Autodesk Inventor part; units mm, degrees
(part 2 of 2)
  spline S316 degree 2 poles (54.544, 56.5341) (54.5622, 56.5549) (54.7827, 56.7857) knots 0 0 0 1 1 1
  spline S317 degree 2 poles (54.7827, 56.7857) (54.6633, 56.8583) (54.5622, 56.9751) (54.5622, 57.0477) knots 0 0 0 1 2 2 2
  spline S318 degree 2 poles (54.5622, 57.0477) (54.5622, 57.1281) (54.6945, 57.3486) (54.9357, 57.5509) knots 0 0 0 1 2 2 2
  spline S319 degree 2 poles (54.9124, 56.7676) (54.8008, 56.6482) (54.6893, 56.4433) (54.6893, 56.3577) knots 0 0 0 1 2 2 2
  spline S320 degree 2 poles (54.6893, 56.3577) (54.6893, 56.2462) (54.8242, 56.1632) knots 0 0 0 1 1 1
  spline S321 degree 2 poles (54.8242, 56.1632) (55.0602, 56.0179) (55.5038, 56.0179) knots 0 0 0 1 1 1
  spline S322 degree 2 poles (55.5038, 56.0179) (55.924, 56.0179) (56.3261, 56.3136) (56.3261, 56.4796) knots 0 0 0 1 2 2 2
  spline S323 degree 2 poles (56.3261, 56.4796) (56.3261, 56.6015) (56.2067, 56.6534) knots 0 0 0 1 1 1
  spline S324 degree 2 poles (56.2067, 56.6534) (56.0848, 56.7027) (55.7243, 56.7131) knots 0 0 0 1 1 1
  spline S325 degree 2 poles (55.7243, 56.7131) (55.1951, 56.7261) (54.9124, 56.7676) knots 0 0 0 1 1 1
  spline S326 degree 2 poles (55.343, 58.8635) (55.1692, 58.8635) (54.9357, 58.5885) (54.9357, 58.3032) knots 0 0 0 1 2 2 2
  spline S327 degree 2 poles (54.9357, 58.3032) (54.9357, 57.9322) (55.0939, 57.7299) knots 0 0 0 1 1 1
  spline S328 degree 2 poles (55.0939, 57.7299) (55.2159, 57.5743) (55.4052, 57.5743) knots 0 0 0 1 1 1
  spline S329 degree 2 poles (55.4052, 57.5743) (55.5816, 57.5743) (55.8125, 57.8415) (55.8125, 58.1268) knots 0 0 0 1 2 2 2
  spline S330 degree 2 poles (55.8125, 58.1268) (55.8125, 58.4977) (55.6516, 58.7078) knots 0 0 0 1 1 1
  spline S331 degree 2 poles (55.6516, 58.7078) (55.5323, 58.8635) (55.343, 58.8635) knots 0 0 0 1 1 1
  line L195 (60.0095, 57.3771) -> (59.7864, 56.7676)
  line L196 (59.7864, 56.7676) -> (57.9136, 56.7676)
  line L197 (57.9136, 56.7676) -> (57.9136, 56.8532)
  spline S332 degree 2 poles (57.9136, 56.8532) (58.741, 57.608) (59.4155, 58.5626) (59.4155, 58.9594) knots 0 0 0 1 2 2 2
  spline S333 degree 2 poles (59.4155, 58.9594) (59.4155, 59.2603) (59.0445, 59.6494) (58.7877, 59.6494) knots 0 0 0 1 2 2 2
  spline S334 degree 2 poles (58.7877, 59.6494) (58.5517, 59.6494) (58.1807, 59.3745) (58.09, 59.1099) knots 0 0 0 1 2 2 2
  line L198 (58.09, 59.1099) -> (58.0044, 59.1099)
  spline S335 degree 2 poles (58.0044, 59.1099) (58.064, 59.5431) (58.5465, 60.0074) (58.9096, 60.0074) knots 0 0 0 1 2 2 2
  spline S336 degree 2 poles (58.9096, 60.0074) (59.2961, 60.0074) (59.8149, 59.512) (59.8149, 59.1747) knots 0 0 0 1 2 2 2
  spline S337 degree 2 poles (59.8149, 59.1747) (59.8149, 58.9335) (59.7034, 58.6923) knots 0 0 0 1 1 1
  spline S338 degree 2 poles (59.7034, 58.6923) (59.5296, 58.3136) (59.1405, 57.8881) knots 0 0 0 1 1 1
  spline S339 degree 2 poles (59.1405, 57.8881) (58.5569, 57.2526) (58.4116, 57.1203) knots 0 0 0 1 1 1
  line L199 (58.4116, 57.1203) -> (59.2417, 57.1203)
  spline S340 degree 2 poles (59.2417, 57.1203) (59.4959, 57.1203) (59.6982, 57.1567) (59.8616, 57.2734) (59.9239, 57.3771) knots 0 0 0 1 2 3 3 3
  line L200 (59.9239, 57.3771) -> (60.0095, 57.3771)
  line L201 (62.3622, 60.0074) -> (62.3622, 59.9218)
  spline S341 degree 2 poles (62.3622, 59.9218) (62.0535, 59.8907) (61.6592, 59.7065) (61.2779, 59.3278) (61.0263, 58.8609) (60.9407, 58.5392) knots 0 0 0 1 2 3 4 4 4
  spline S342 degree 2 poles (60.9407, 58.5392) (61.2805, 58.7727) (61.6203, 58.7727) knots 0 0 0 1 1 1
  spline S343 degree 2 poles (61.6203, 58.7727) (61.9446, 58.7727) (62.4245, 58.2487) (62.4245, 57.8363) knots 0 0 0 1 2 2 2
  spline S344 degree 2 poles (62.4245, 57.8363) (62.4245, 57.4394) (62.1832, 57.11) knots 0 0 0 1 1 1
  spline S345 degree 2 poles (62.1832, 57.11) (61.8927, 56.7131) (61.4128, 56.7131) knots 0 0 0 1 1 1
  spline S346 degree 2 poles (61.4128, 56.7131) (61.0886, 56.7131) (60.8603, 56.9284) knots 0 0 0 1 1 1
  spline S347 degree 2 poles (60.8603, 56.9284) (60.4141, 57.346) (60.4141, 58.0152) knots 0 0 0 1 1 1
  spline S348 degree 2 poles (60.4141, 58.0152) (60.4141, 58.4407) (60.7565, 59.2085) (61.3921, 59.8025) (61.9757, 60.0074) (62.2273, 60.0074) knots 0 0 0 1 2 3 4 4 4
  line L202 (62.2273, 60.0074) -> (62.3622, 60.0074)
  spline S349 degree 2 poles (60.9018, 58.368) (60.8603, 58.0542) (60.8603, 57.8596) knots 0 0 0 1 1 1
  spline S350 degree 2 poles (60.8603, 57.8596) (60.8603, 57.6365) (61.0263, 57.11) (61.1897, 56.9543) knots 0 0 0 1 2 2 2
  spline S351 degree 2 poles (61.1897, 56.9543) (61.3116, 56.8454) (61.4829, 56.8454) knots 0 0 0 1 1 1
  spline S352 degree 2 poles (61.4829, 56.8454) (61.6852, 56.8454) (62.0068, 57.2293) (62.0068, 57.5847) knots 0 0 0 1 2 2 2
  spline S353 degree 2 poles (62.0068, 57.5847) (62.0068, 57.9841) (61.6878, 58.5678) (61.3947, 58.5678) knots 0 0 0 1 2 2 2
  spline S354 degree 2 poles (61.3947, 58.5678) (61.3065, 58.5678) (61.1015, 58.4925) (60.9018, 58.368) knots 0 0 0 1 2 2 2
  line L203 (63.3842, 59.6183) -> (63.3842, 58.9128)
  line L204 (63.3842, 58.9128) -> (63.8849, 58.9128)
  line L205 (63.8849, 58.9128) -> (63.8849, 58.7493)
  line L206 (63.8849, 58.7493) -> (63.3842, 58.7493)
  line L207 (63.3842, 58.7493) -> (63.3842, 57.3564)
  spline S355 degree 2 poles (63.3842, 57.3564) (63.3842, 57.1489) (63.5035, 57.0036) (63.5969, 57.0036) knots 0 0 0 1 2 2 2
  spline S356 degree 2 poles (63.5969, 57.0036) (63.6747, 57.0036) (63.8226, 57.0996) (63.8615, 57.193) knots 0 0 0 1 2 2 2
  line L208 (63.8615, 57.193) -> (63.9523, 57.193)
  spline S357 degree 2 poles (63.9523, 57.193) (63.8693, 56.9621) (63.5684, 56.7312) (63.4102, 56.7312) knots 0 0 0 1 2 2 2
  spline S358 degree 2 poles (63.4102, 56.7312) (63.3012, 56.7312) (63.0937, 56.8506) (62.9951, 57.0736) (62.9951, 57.3045) knots 0 0 0 1 2 3 3 3
  line L209 (62.9951, 57.3045) -> (62.9951, 58.7493)
  line L210 (62.9951, 58.7493) -> (62.6553, 58.7493)
  line L211 (62.6553, 58.7493) -> (62.6553, 58.8272)
  spline S359 degree 2 poles (62.6553, 58.8272) (62.785, 58.879) (63.0548, 59.1229) (63.1611, 59.2915) knots 0 0 0 1 2 2 2
  spline S360 degree 2 poles (63.1611, 59.2915) (63.2156, 59.3823) (63.3116, 59.6183) knots 0 0 0 1 1 1
  line L212 (63.3116, 59.6183) -> (63.3842, 59.6183)
  line L213 (64.7227, 60.0982) -> (64.7227, 58.5289)
  spline S361 degree 2 poles (64.7227, 58.5289) (64.9821, 58.8142) (65.2856, 58.975) (65.4386, 58.975) knots 0 0 0 1 2 2 2
  spline S362 degree 2 poles (65.4386, 58.975) (65.6202, 58.975) (65.8848, 58.7727) (65.947, 58.5574) knots 0 0 0 1 2 2 2
  spline S363 degree 2 poles (65.947, 58.5574) (65.9911, 58.4095) (65.9911, 58.0101) knots 0 0 0 1 1 1
  line L214 (65.9911, 58.0101) -> (65.9911, 57.2526)
  spline S364 degree 2 poles (65.9911, 57.2526) (65.9911, 57.0503) (66.0249, 56.9751) knots 0 0 0 1 1 1
  spline S365 degree 2 poles (66.0249, 56.9751) (66.0482, 56.918) (66.1598, 56.8532) (66.3102, 56.8532) knots 0 0 0 1 2 2 2
  line L215 (66.3102, 56.8532) -> (66.3102, 56.7676)
  line L216 (66.3102, 56.7676) -> (65.2545, 56.7676)
  line L217 (65.2545, 56.7676) -> (65.2545, 56.8532)
  line L218 (65.2545, 56.8532) -> (65.3037, 56.8532)
  spline S366 degree 2 poles (65.3037, 56.8532) (65.4542, 56.8532) (65.5709, 56.9439) (65.5943, 57.0321) knots 0 0 0 1 2 2 2
  spline S367 degree 2 poles (65.5943, 57.0321) (65.6021, 57.0711) (65.6021, 57.2526) knots 0 0 0 1 1 1
  line L219 (65.6021, 57.2526) -> (65.6021, 58.0101)
  spline S368 degree 2 poles (65.6021, 58.0101) (65.6021, 58.3628) (65.5294, 58.5833) (65.3712, 58.6923) (65.2571, 58.6923) knots 0 0 0 1 2 3 3 3
  spline S369 degree 2 poles (65.2571, 58.6923) (65.1429, 58.6923) (64.8965, 58.5704) (64.7227, 58.3862) knots 0 0 0 1 2 2 2
  line L220 (64.7227, 58.3862) -> (64.7227, 57.2526)
  spline S370 degree 2 poles (64.7227, 57.2526) (64.7227, 57.0321) (64.772, 56.9258) (64.9069, 56.8532) (65.0703, 56.8532) knots 0 0 0 1 2 3 3 3
  line L221 (65.0703, 56.8532) -> (65.0703, 56.7676)
  line L222 (65.0703, 56.7676) -> (64.0068, 56.7676)
  line L223 (64.0068, 56.7676) -> (64.0068, 56.8532)
  spline S371 degree 2 poles (64.0068, 56.8532) (64.1494, 56.8532) (64.2298, 56.8973) knots 0 0 0 1 1 1
  spline S372 degree 2 poles (64.2298, 56.8973) (64.2765, 56.9206) (64.3336, 57.0529) (64.3336, 57.2526) knots 0 0 0 1 2 2 2
  line L224 (64.3336, 57.2526) -> (64.3336, 59.1955)
  spline S373 degree 2 poles (64.3336, 59.1955) (64.3336, 59.5612) (64.2973, 59.7273) (64.2247, 59.7869) (64.165, 59.7869) knots 0 0 0 1 2 3 3 3
  spline S374 degree 2 poles (64.165, 59.7869) (64.1157, 59.7869) (64.0068, 59.7506) knots 0 0 0 1 1 1
  line L225 (64.0068, 59.7506) -> (63.973, 59.8362)
  line L226 (63.973, 59.8362) -> (64.6138, 60.0982)
  line L227 (64.6138, 60.0982) -> (64.7227, 60.0982)
  line L228 (69.7394, 57.3771) -> (69.5163, 56.7676)
  line L229 (69.5163, 56.7676) -> (67.6435, 56.7676)
  line L230 (67.6435, 56.7676) -> (67.6435, 56.8532)
  spline S375 degree 2 poles (67.6435, 56.8532) (68.471, 57.608) (69.1454, 58.5626) (69.1454, 58.9594) knots 0 0 0 1 2 2 2
  spline S376 degree 2 poles (69.1454, 58.9594) (69.1454, 59.2603) (68.7745, 59.6494) (68.5177, 59.6494) knots 0 0 0 1 2 2 2
  spline S377 degree 2 poles (68.5177, 59.6494) (68.2816, 59.6494) (67.9107, 59.3745) (67.8199, 59.1099) knots 0 0 0 1 2 2 2
  line L231 (67.8199, 59.1099) -> (67.7343, 59.1099)
  spline S378 degree 2 poles (67.7343, 59.1099) (67.7939, 59.5431) (68.2764, 60.0074) (68.6396, 60.0074) knots 0 0 0 1 2 2 2
  spline S379 degree 2 poles (68.6396, 60.0074) (69.0261, 60.0074) (69.5449, 59.512) (69.5449, 59.1747) knots 0 0 0 1 2 2 2
  spline S380 degree 2 poles (69.5449, 59.1747) (69.5449, 58.9335) (69.4333, 58.6923) knots 0 0 0 1 1 1
  spline S381 degree 2 poles (69.4333, 58.6923) (69.2595, 58.3136) (68.8704, 57.8881) knots 0 0 0 1 1 1
  spline S382 degree 2 poles (68.8704, 57.8881) (68.2868, 57.2526) (68.1415, 57.1203) knots 0 0 0 1 1 1
  line L232 (68.1415, 57.1203) -> (68.9716, 57.1203)
  spline S383 degree 2 poles (68.9716, 57.1203) (69.2258, 57.1203) (69.4281, 57.1567) (69.5916, 57.2734) (69.6538, 57.3771) knots 0 0 0 1 2 3 3 3
  line L233 (69.6538, 57.3771) -> (69.7394, 57.3771)
  spline S384 degree 2 poles (70.1129, 58.3369) (70.1129, 58.879) (70.4398, 59.6624) (70.7121, 59.8544) knots 0 0 0 1 2 2 2
  spline S385 degree 2 poles (70.7121, 59.8544) (70.9223, 60.0074) (71.1479, 60.0074) knots 0 0 0 1 1 1
  spline S386 degree 2 poles (71.1479, 60.0074) (71.5137, 60.0074) (71.8042, 59.6365) knots 0 0 0 1 1 1
  spline S387 degree 2 poles (71.8042, 59.6365) (72.1673, 59.1747) (72.1673, 58.3862) knots 0 0 0 1 1 1
  spline S388 degree 2 poles (72.1673, 58.3862) (72.1673, 57.8337) (71.8483, 57.0607) (71.3554, 56.7131) (71.1246, 56.7131) knots 0 0 0 1 2 3 3 3
  spline S389 degree 2 poles (71.1246, 56.7131) (70.6706, 56.7131) (70.3671, 57.25) knots 0 0 0 1 1 1
  spline S390 degree 2 poles (70.3671, 57.25) (70.1129, 57.7014) (70.1129, 58.3369) knots 0 0 0 1 1 1
  spline S391 degree 2 poles (70.5721, 58.2772) (70.5721, 57.6236) (70.7329, 57.2085) knots 0 0 0 1 1 1
  spline S392 degree 2 poles (70.7329, 57.2085) (70.8678, 56.8609) (71.1324, 56.8609) knots 0 0 0 1 1 1
  spline S393 degree 2 poles (71.1324, 56.8609) (71.2595, 56.8609) (71.5292, 57.0866) (71.5993, 57.3538) knots 0 0 0 1 2 2 2
  spline S394 degree 2 poles (71.5993, 57.3538) (71.7082, 57.7559) (71.7082, 58.4873) knots 0 0 0 1 1 1
  spline S395 degree 2 poles (71.7082, 58.4873) (71.7082, 59.0321) (71.5967, 59.3926) knots 0 0 0 1 1 1
  spline S396 degree 2 poles (71.5967, 59.3926) (71.5111, 59.6624) (71.3788, 59.774) knots 0 0 0 1 1 1
  spline S397 degree 2 poles (71.3788, 59.774) (71.2828, 59.8518) (71.1453, 59.8518) knots 0 0 0 1 1 1
  spline S398 degree 2 poles (71.1453, 59.8518) (70.9871, 59.8518) (70.8626, 59.7091) knots 0 0 0 1 1 1
  spline S399 degree 2 poles (70.8626, 59.7091) (70.694, 59.5146) (70.5721, 58.6819) (70.5721, 58.2772) knots 0 0 0 1 2 2 2
  line L234 (74.5382, 57.3771) -> (74.3151, 56.7676)
  line L235 (74.3151, 56.7676) -> (72.4423, 56.7676)
  line L236 (72.4423, 56.7676) -> (72.4423, 56.8532)
  spline S400 degree 2 poles (72.4423, 56.8532) (73.2698, 57.608) (73.9442, 58.5626) (73.9442, 58.9594) knots 0 0 0 1 2 2 2
  spline S401 degree 2 poles (73.9442, 58.9594) (73.9442, 59.2603) (73.5733, 59.6494) (73.3165, 59.6494) knots 0 0 0 1 2 2 2
  spline S402 degree 2 poles (73.3165, 59.6494) (73.0804, 59.6494) (72.7095, 59.3745) (72.6187, 59.1099) knots 0 0 0 1 2 2 2
  line L237 (72.6187, 59.1099) -> (72.5331, 59.1099)
  spline S403 degree 2 poles (72.5331, 59.1099) (72.5928, 59.5431) (73.0752, 60.0074) (73.4384, 60.0074) knots 0 0 0 1 2 2 2
  spline S404 degree 2 poles (73.4384, 60.0074) (73.8249, 60.0074) (74.3437, 59.512) (74.3437, 59.1747) knots 0 0 0 1 2 2 2
  spline S405 degree 2 poles (74.3437, 59.1747) (74.3437, 58.9335) (74.2321, 58.6923) knots 0 0 0 1 1 1
  spline S406 degree 2 poles (74.2321, 58.6923) (74.0583, 58.3136) (73.6692, 57.8881) knots 0 0 0 1 1 1
  spline S407 degree 2 poles (73.6692, 57.8881) (73.0856, 57.2526) (72.9403, 57.1203) knots 0 0 0 1 1 1
  line L238 (72.9403, 57.1203) -> (73.7704, 57.1203)
  spline S408 degree 2 poles (73.7704, 57.1203) (74.0246, 57.1203) (74.2269, 57.1567) (74.3904, 57.2734) (74.4526, 57.3771) knots 0 0 0 1 2 3 3 3
  line L239 (74.4526, 57.3771) -> (74.5382, 57.3771)
  line L240 (76.8209, 59.9426) -> (76.6393, 59.5457)
  line L241 (76.6393, 59.5457) -> (75.6848, 59.5457)
  line L242 (75.6848, 59.5457) -> (75.4746, 59.1203)
  spline S409 degree 2 poles (75.4746, 59.1203) (76.0946, 59.0295) (76.4577, 58.6586) knots 0 0 0 1 1 1
  spline S410 degree 2 poles (76.4577, 58.6586) (76.769, 58.3395) (76.769, 57.9089) knots 0 0 0 1 1 1
  spline S411 degree 2 poles (76.769, 57.9089) (76.769, 57.6599) (76.5641, 57.2319) (76.2554, 56.9336) (76.0661, 56.8428) knots 0 0 0 1 2 3 3 3
  spline S412 degree 2 poles (76.0661, 56.8428) (75.7963, 56.7131) (75.5135, 56.7131) knots 0 0 0 1 1 1
  spline S413 degree 2 poles (75.5135, 56.7131) (75.2256, 56.7131) (74.9662, 56.9076) (74.9662, 57.0244) knots 0 0 0 1 2 2 2
  spline S414 degree 2 poles (74.9662, 57.0244) (74.9662, 57.0892) (75.0726, 57.1904) (75.1556, 57.1904) knots 0 0 0 1 2 2 2
  spline S415 degree 2 poles (75.1556, 57.1904) (75.2152, 57.1904) (75.3086, 57.1515) (75.4176, 57.0736) knots 0 0 0 1 2 2 2
  spline S416 degree 2 poles (75.4176, 57.0736) (75.594, 56.9543) (75.7755, 56.9517) knots 0 0 0 1 1 1
  spline S417 degree 2 poles (75.7755, 56.9517) (76.0479, 56.9517) (76.4655, 57.3668) (76.4655, 57.6651) knots 0 0 0 1 2 2 2
  spline S418 degree 2 poles (76.4655, 57.6651) (76.4655, 57.953) (76.0946, 58.4536) (75.7678, 58.5885) knots 0 0 0 1 2 2 2
  spline S419 degree 2 poles (75.7678, 58.5885) (75.5135, 58.6949) (75.0726, 58.7104) knots 0 0 0 1 1 1
  line L243 (75.0726, 58.7104) -> (75.6822, 59.9426)
  line L244 (75.6822, 59.9426) -> (76.8209, 59.9426)
  point P0 (0, 120.8)
  dimension "d0" = 191.4
  dimension "d1" = 121.8
  constraints: 2 other
emboss "Emboss2" sketch "Sketch9" operation cut depth 1 direction (0, 1, 0)
sketch "Sketch10" plane through (0, 0, -120.8) normal (0, -1, 0) x (1, 0, 0)
  point P0 (0, 120.8)
sketch "Sketch11" plane through (0, 0, -120.8) normal (0, -1, 0) x (1, 0, 0)
  point P0 (0, 120.8)
sketch "Sketch13" plane through (110, 12.5, -116.4021) normal (1, 0, 0) x (0, 0, -1)
  point P0 (-116.4021, -12.5)
sketch "Sketch14" plane through (110, 12.5, -116.4021) normal (1, 0, 0) x (0, 0, -1)
  point P0 (-116.4021, -12.5)
ref_plane "Work Plane1" through (111, 12.5, -116.4021) normal (1, 0, 0) x (0, 0, -1)
sketch "Sketch16" plane through (111, 12.5, -116.4021) normal (1, 0, 0) x (0, 0, -1)
  arc A0 (-4, 14.7262) -> (-4, 9.7262) centre (-4, 12.2262) ccw
  line L0 (0, 178.9) -> (0, 0) projected
  line L1 (-4, 14.7262) -> (-4, 9.7262)
  point P0 (-116.4021, -12.5)
  dimension "d27" = 5
  dimension "d28" = 4
  constraints: 2 end point, 2 point on circle, 1 centre point, 1 vertical
  measures "d27" diameter of A0
  measures "d28" distance from line of A0.centre L0
revolve "Revolution2" cut sketch "Sketch16" angle 360 about axis through (111, 27.2262, -112.4021) along (0, -1, 0)
sketch "Sketch17" plane through (111, 12.5, -116.4021) normal (1, 0, 0) x (0, 0, -1)
  point P0 (-116.4021, -12.5)
sketch "Sketch18" plane through (111, 12.5, -116.4021) normal (1, 0, 0) x (0, 0, -1)
  arc A0 (-107.0042, 14.736) -> (-107.0042, 9.736) centre (-107.0042, 12.236) ccw
  line L0 (-111.0042, 178.9) -> (-111.0042, 0) projected
  line L1 (-111.0042, 0) -> (-104.0021, 0) projected
  line L2 (-107.0042, 14.736) -> (-107.0042, 9.736)
  point P0 (-116.4021, -12.5)
  dimension "d30" = 5
  dimension "d31" = 4
  dimension "d32" = 12.236
  constraints: 2 end point, 2 point on circle, 1 centre point, 1 parallel
  measures "d30" diameter of A0
  measures "d31" distance from line of A0.centre L0
  measures "d32" distance from line of A0.centre L1
revolve "Revolution3" cut sketch "Sketch18" angle 360 about axis through (111, 27.236, -9.3979) along (0, -1, 0)
sketch "Sketch19" plane through (110, 12.5, -116.4021) normal (1, 0, 0) x (0, 0, -1)
  point P0 (-116.4021, -12.5)
sketch "Sketch20" plane through (110, 12.5, -116.4021) normal (1, 0, 0) x (0, 0, -1)
  line L0 (-104.0021, 166.4) -> (-7.0021, 166.4) projected
  line L1 (-104.0021, 0) -> (-104.0021, 178.9) projected
  line L2 (-7.0021, 166.4) -> (-104.0021, 166.4)
  line L3 (-104.0021, 166.4) -> (-104.0021, 168.4)
  line L4 (-104.0021, 168.4) -> (-7.0021, 168.4)
  line L5 (-7.0021, 168.4) -> (-7.0021, 166.4)
  point P0 (-116.4021, -12.5)
  dimension "d34" = 2
  constraints: 8 end point, 2 parallel, 1 horizontal, 1 perpendicular, 1 point on line
  measures "d34" distance between parallel lines of L4 L0
extrude "Extrusion5" cut sketch "Sketch20" against normal up to surface (95 mm away)
sketch "Sketch21" plane through (110, 12.5, -116.4021) normal (1, 0, 0) x (0, 0, -1)
  line L0 (-7.0021, 168.4) -> (-7.0021, 0) projected
  line L1 (-7.0021, 0) -> (-6.4021, 0)
  line L2 (-6.4021, 0) -> (-6.4021, 168.4)
  line L3 (-6.4021, 168.4) -> (-7.0021, 168.4)
  line L4 (-7.0021, 168.4) -> (-7.0021, 0)
  point P0 (-116.4021, -12.5)
  dimension "d37" = 0.6
  constraints: 8 end point, 2 parallel, 1 horizontal, 1 perpendicular
  measures "d37" distance between parallel lines of L0 L2
sketch "Sketch22" plane through (110, 12.5, -116.4021) normal (1, 0, 0) x (0, 0, -1)
  line L0 (-104.0021, 0) -> (-104.6021, 0)
  line L1 (-104.6021, 0) -> (-104.6021, 168.4)
  line L2 (-104.6021, 168.4) -> (-104.0021, 168.4)
  line L3 (-104.0021, 168.4) -> (-104.0021, 0)
  point P0 (-116.4021, -12.5)
  dimension "d38" = 0.6
  constraints: 8 end point, 2 parallel, 1 horizontal, 1 perpendicular
  measures "d38" distance between parallel lines of L3 L1
extrude "Extrusion6" cut sketch "Sketch22" against normal up to surface (95 mm away)
extrude "Extrusion7" cut sketch "Sketch21" against normal up to surface (95 mm away)
sketch "Sketch23" plane through (110, 12.5, -116.4021) normal (1, 0, 0) x (0, 0, -1)
  line L0 (-104.6021, 168.4) -> (-6.4021, 168.4)
  line L1 (-6.4021, 168.4) -> (-6.4021, 169.4)
  line L2 (-6.4021, 169.4) -> (-104.6021, 169.4)
  line L3 (-104.6021, 169.4) -> (-104.6021, 168.4)
  point P0 (-116.4021, -12.5)
  dimension "d43" = 1
  constraints: 8 end point, 2 parallel, 1 horizontal, 1 perpendicular
  measures "d43" distance between parallel lines of L2 L0
extrude "Extrusion8" cut sketch "Sketch23" against normal up to surface (95 mm away)
body "Solid1"
